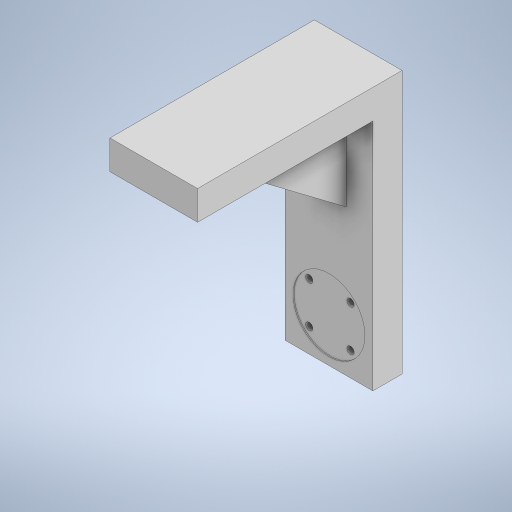
# Autodesk Inventor part: EndEffectorMotorAdapterOLD
Saved by Autodesk Inventor 2024 (Build 280153000, 153)
## iProperties
Created: 2024-02-13
Part Number: EndEffectorMotorAdapterOLD
Material: Generic
Document SubType Name: Modeling
Designer: yusuf
Density: 1 g/cm^3
Appearance: Default
Author: yusuf
Autodesk Inventor part; units mm, degrees
ref_plane "YZ Plane" through (0, 0, 0) normal (1, 0, 0) x (0, 1, 0)
ref_plane "XZ Plane" through (0, 0, 0) normal (0, 1, 0) x (-1, 0, 0)
ref_plane "XY Plane" through (0, 0, 0) normal (0, 0, 1) x (1, 0, 0)
sketch "Sketch7" plane through (0, 0, 0) normal (0, 0, 1) x (1, 0, 0)
  circle A0 centre (0, 0) radius 31.2801
  dimension "d33" = 62.5602
  constraints: 1 centre point, 1 coincident
  measures "d33" diameter of A0
extrude "Extrusion8" add sketch "Sketch7" along normal blind 50
sketch "Sketch9" plane through (0, 0, 0) normal (0, 0, -1) x (-1, 0, 0)
  line L0 (-38.1, 38.1) -> (38.1, 38.1)
  line L1 (38.1, 38.1) -> (38.1, -38.1)
  line L2 (38.1, -38.1) -> (-38.1, -38.1)
  line L3 (-38.1, -38.1) -> (-38.1, 38.1)
  line L4 (-38.1, 38.1) -> (38.1, -38.1) construction
  line L5 (38.1, 38.1) -> (-38.1, -38.1) construction
  point P0 (0, 0)
  dimension "d43" = 76.2
  dimension "d44" = 76.2
  constraints: 12 end point, 2 midpoint, 2 parallel, 1 horizontal, 1 perpendicular
  measures "d43" distance of L0.end L1.end
  measures "d44" distance of L1.end L2.end
extrude "Extrusion10" add sketch "Sketch9" along normal blind 25.4
sketch "Sketch10" plane through (-38.1, 38.1, 0) normal (0, 1, 0) x (1, 0, 0)
  line L0 (76.2, 0) -> (0, 0) projected
  line L1 (76.2, 0) -> (76.2, 25.4) projected
  line L2 (0, 0) -> (76.2, 0)
  line L3 (76.2, 0) -> (76.2, 25.4)
  line L4 (76.2, 25.4) -> (0, 25.4)
  line L5 (0, 25.4) -> (0, 0)
  point P0 (38.1, 0)
  constraints: 8 end point, 2 parallel, 1 horizontal, 1 perpendicular
extrude "Extrusion11" add sketch "Sketch10" along normal blind 152.4
sketch "Sketch11" plane through (0, 0, 0) normal (0, 0, 1) x (1, 0, 0)
  line L0 (-38.1, -38.1) -> (-38.1, 190.5) projected
  line L1 (38.1, -38.1) -> (38.1, 190.5) projected
  line L2 (-38.1, 190.5) -> (38.1, 190.5)
  line L3 (38.1, 190.5) -> (38.1, 165.1)
  line L4 (38.1, 165.1) -> (-38.1, 165.1)
  line L5 (-38.1, 165.1) -> (-38.1, 190.5)
  point P0 (0, 0)
  point P1 (-38.1, 165.1)
  dimension "d49" = 25.4
  constraints: 8 end point, 2 parallel, 1 horizontal, 1 perpendicular, 1 point on line
  measures "d49" distance between parallel lines of L2 L4
extrude "Extrusion12" add sketch "Sketch11" along normal blind 152.4
sketch "Sketch14" plane through (0, 0, 0) normal (1, 0, 0) x (0, 1, 0)
  line L0 (-38.1, 0) -> (165.1, 0) projected
  line L1 (165.1, 0) -> (88.9, 0)
  line L2 (-38.1, 0) -> (165.1, 0) projected
  line L3 (88.9, 0) -> (165.4611, 101.6)
  point P0 (0, 0)
  dimension "d70" = 76.2
  dimension "d71" = -53
  dimension "d72" = 101.6
  constraints: 4 end point, 1 point on line
  measures "d70" distance of L0.end L1.end
  measures "d71" angle of L0 L3
  measures "d72" distance from line of L3.end L2
extrude "Rib2" add sketch "Sketch14" along normal mid plane 30 rib yes fills toward (127, 0.05) open curves L1 L3
sketch "Sketch16" plane through (0, 0, 50) normal (0, 0, 1) x (1, 0, 0)
  circle A0 centre (17.9578, -17.9578) radius 3.175
  circle A1 centre (17.9578, 17.9578) radius 3.175
  circle A2 centre (-17.9578, 17.9578) radius 3.175
  circle A3 centre (-17.9578, -17.9578) radius 3.175
  point P0 (0, 0)
  dimension "d89" = 6.35
  dimension "d90" = 17.9578
  dimension "d91" = 17.9578
  dimension "d94" = 360
  constraints: 4 centre point, 9 other
  measures "d89" diameter of A0
  measures "d90" horizontal distance of point (0, 0) A0.centre
  measures "d91" horizontal distance of point (0, 0) A0.centre
extrude "Extrusion14" cut sketch "Sketch16" against normal through all
sketch "Sketch17" plane through (0, 0, 50) normal (0, 0, 1) x (1, 0, 0)
  circle A0 centre (0, 0) radius 31.2801
  circle A1 centre (0, 0) radius 31.2801 projected
  dimension "d98" = 0
  constraints: 1 centre point, 1 coincident
  measures "d98" radial gap between concentric circles of A1 A0
extrude "Extrusion15" cut sketch "Sketch17" against normal blind 50.8
body "Solid2"
